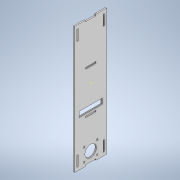
# Autodesk Inventor part: MuurL
Saved by Autodesk Inventor 2020 (Build 240168000, 168)
## iProperties
Created: 2020-01-30
Part Number: MuurL
Material: Generic
Document SubType Name: Modeling
Designer: jelte
Density: 1 g/cm^3
Appearance: Default
Mass: 62.7355 g
Surface Area: 455.02 cm^2
Volume: 62.7355 cm^3
Author: jelte
Autodesk Inventor part; units mm, degrees
ref_plane "YZ Plane" through (0, 0, 0) normal (1, 0, 0) x (0, 1, 0)
ref_plane "XZ Plane" through (0, 0, 0) normal (0, 1, 0) x (-1, 0, 0)
ref_plane "XY Plane" through (0, 0, 0) normal (0, 0, 1) x (1, 0, 0)
sketch "Sketch1" plane through (0, 0, 0) normal (1, 0, 0) x (0, 1, 0)
  line L0 (136.2492, 38.7083) -> (-163.7508, 38.7083)
  line L1 (-163.7508, -36.2917) -> (136.2492, -36.2917)
  line L2 (-160.7508, 13.7083) -> (-160.7508, -11.2917)
  line L3 (-160.7508, -11.2917) -> (-163.7508, -11.2917)
  line L4 (-160.7508, 13.7083) -> (-163.7508, 13.7083)
  line L5 (-163.7508, 13.7083) -> (-163.7508, 38.7083)
  line L6 (-163.7508, -11.2917) -> (-163.7508, -36.2917)
  line L7 (136.2492, 38.7083) -> (136.2492, 13.7083)
  line L8 (136.2492, -36.2917) -> (136.2492, -11.2917)
  line L9 (136.2492, 13.7083) -> (133.2492, 13.7083)
  line L10 (133.2492, 13.7083) -> (133.2492, -11.2917)
  line L11 (136.2492, -11.2917) -> (133.2492, -11.2917)
  point P0 (0, 0)
  dimension "d1" = 300
  constraints: 24 end point, 4 vertical, 2 equal length, 2 horizontal, 1 perpendicular
  measures "d1" distance of L1.start L1.end
extrude "Extrusion1" add sketch "Sketch1" along normal blind 3
sketch "Sketch2" plane through (3, 0, 0) normal (1, 0, 0) x (0, 0, -1)
  line L0 (-13.7083, -163.7508) -> (-13.7083, -160.7508) projected
  line L1 (-13.7083, -160.7508) -> (11.2917, -160.7508) projected
  line L2 (-13.7083, -60.7508) -> (11.2917, -60.7508)
  line L3 (11.2917, -60.7508) -> (11.2917, -63.7508)
  line L4 (11.2917, -63.7508) -> (-13.7083, -63.7508)
  line L5 (-13.7083, -63.7508) -> (-13.7083, -60.7508)
  line L6 (36.2917, -163.7508) -> (36.2917, 136.2492) projected
  line L7 (-13.7083, 36.2492) -> (11.2917, 36.2492)
  line L8 (11.2917, 36.2492) -> (11.2917, 39.2492)
  line L9 (11.2917, 39.2492) -> (-13.7083, 39.2492)
  line L10 (-13.7083, 39.2492) -> (-13.7083, 36.2492)
  point P0 (0, 0)
  constraints: 16 end point, 4 parallel, 2 horizontal, 2 perpendicular
extrude "Extrusion2" cut sketch "Sketch2" against normal blind 3
sketch "Sketch3" plane through (3, 0, 0) normal (1, 0, 0) x (0, 0, -1)
  line L0 (-13.7083, -160.7508) -> (11.2917, -160.7508) projected
  circle A0 centre (-16.7083, -154.7508) radius 1.5
  circle A1 centre (14.2917, -154.7508) radius 1.5
  circle A2 centre (14.2917, -123.7508) radius 1.5
  circle A3 centre (-16.7083, -123.7508) radius 1.5
  circle A4 centre (-1.2083, -139.2508) radius 12
  point P0 (0, 0)
  dimension "d29" = 3
  dimension "d30" = 3
  dimension "d31" = 3
  dimension "d32" = 3
  dimension "d33" = 24
  constraints: 5 centre point
  measures "d29" diameter of A2
  measures "d30" diameter of A3
  measures "d31" diameter of A0
  measures "d32" diameter of A1
  measures "d33" diameter of A4
extrude "Extrusion3" cut sketch "Sketch3" against normal blind 3
sketch "Sketch4" plane through (3, 0, 0) normal (1, 0, 0) x (0, 0, -1)
  line L0 (-13.7083, -160.7508) -> (11.2917, -160.7508) projected
  line L1 (36.2917, -163.7508) -> (36.2917, 136.2492) projected
  line L2 (31.2917, -155.7508) -> (28.2917, -155.7508)
  line L3 (28.2917, -155.7508) -> (28.2917, -145.7508)
  line L4 (28.2917, -145.7508) -> (31.2917, -145.7508)
  line L5 (31.2917, -145.7508) -> (31.2917, -155.7508)
  line L6 (-38.7083, 136.2492) -> (-38.7083, -163.7508) projected
  line L7 (-33.7083, -155.7508) -> (-30.7083, -155.7508)
  line L8 (-30.7083, -155.7508) -> (-30.7083, -145.7508)
  line L9 (-30.7083, -145.7508) -> (-33.7083, -145.7508)
  line L10 (-33.7083, -145.7508) -> (-33.7083, -155.7508)
  line L11 (-33.7083, 128.1373) -> (-30.7083, 128.1373)
  line L12 (-30.7083, 128.1373) -> (-30.7083, 118.1373)
  line L13 (-30.7083, 118.1373) -> (-33.7083, 118.1373)
  line L14 (-33.7083, 118.1373) -> (-33.7083, 128.1373)
  line L15 (31.2917, 128.1373) -> (28.2917, 128.1373)
  line L16 (28.2917, 128.1373) -> (28.2917, 118.1373)
  line L17 (28.2917, 118.1373) -> (31.2917, 118.1373)
  line L18 (31.2917, 118.1373) -> (31.2917, 128.1373)
  point P0 (0, 0)
  dimension "d38" = 3
  dimension "d39" = 10
  dimension "d46" = 3
  dimension "d47" = 10
  dimension "d48" = 3
  dimension "d49" = 10
  dimension "d50" = 10
  dimension "d51" = 3
  constraints: 32 end point, 8 parallel, 4 horizontal, 4 perpendicular
  measures "d38" distance of L3.end L4.end
  measures "d39" distance of L4.end L2.start
  measures "d46" distance of L8.end L9.end
  measures "d47" distance of L7.end L8.end
  measures "d48" distance of L12.end L13.end
  measures "d49" distance of L11.end L12.end
  measures "d50" distance of L15.end L16.end
  measures "d51" distance of L16.end L17.end
extrude "Extrusion4" cut sketch "Sketch4" against normal blind 30
sketch "Sketch5" plane through (3, 0, 0) normal (1, 0, 0) x (0, 0, -1)
  line L0 (-13.7083, -60.7508) -> (11.2917, -60.7508) projected
  line L1 (-38.7083, 136.2492) -> (-38.7083, -163.7508) projected
  line L2 (36.2917, -163.7508) -> (36.2917, 136.2492) projected
  line L3 (-28.7083, -55.7508) -> (26.2917, -55.7508)
  line L4 (26.2917, -55.7508) -> (26.2917, -43.2508)
  line L5 (26.2917, -43.2508) -> (-28.7083, -43.2508)
  line L6 (-28.7083, -43.2508) -> (-28.7083, -55.7508)
  point P0 (0, 0)
  constraints: 8 end point, 2 parallel, 1 horizontal, 1 perpendicular
extrude "Extrusion5" cut sketch "Sketch5" against normal blind 10
sketch "Sketch6" plane through (3, 0, 0) normal (1, 0, 0) x (0, 0, -1)
  line L0 (-30.7083, 118.1373) -> (-33.7083, 118.1373) projected
  line L1 (-33.7083, 118.1373) -> (-30.7083, 118.1373)
  line L2 (-30.7083, 118.1373) -> (-30.7083, 103.1373)
  line L3 (-30.7083, 103.1373) -> (-33.7083, 103.1373)
  line L4 (-33.7083, 103.1373) -> (-33.7083, 118.1373)
  line L5 (28.2917, 118.1373) -> (31.2917, 118.1373) projected
  line L6 (28.2917, 118.1373) -> (31.2917, 118.1373)
  line L7 (31.2917, 118.1373) -> (31.2917, 103.1373)
  line L8 (31.2917, 103.1373) -> (28.2917, 103.1373)
  line L9 (28.2917, 103.1373) -> (28.2917, 118.1373)
  line L10 (-33.7083, -155.7508) -> (-33.7083, -145.7508) projected
  line L11 (-33.7083, -145.7508) -> (-30.7083, -145.7508)
  line L12 (-30.7083, -145.7508) -> (-30.7083, -130.7508)
  line L13 (-30.7083, -130.7508) -> (-33.7083, -130.7508)
  line L14 (-33.7083, -130.7508) -> (-33.7083, -145.7508)
  line L15 (28.2917, -155.7508) -> (28.2917, -145.7508) projected
  line L16 (28.2917, -145.7508) -> (31.2917, -145.7508)
  line L17 (31.2917, -145.7508) -> (31.2917, -130.7508)
  line L18 (31.2917, -130.7508) -> (28.2917, -130.7508)
  line L19 (28.2917, -130.7508) -> (28.2917, -145.7508)
  point P0 (0, 0)
  dimension "d62" = 15
  dimension "d63" = 15
  constraints: 32 end point, 8 parallel, 4 horizontal, 4 perpendicular
  measures "d62" distance of L11.end L12.end
  measures "d63" distance of L16.end L17.end
extrude "Extrusion6" cut sketch "Sketch6" against normal blind 10
sketch "Sketch7" plane through (3, 0, 0) normal (1, 0, 0) x (0, 0, -1)
  point P0 (0, 0)
sketch "Sketch8" plane through (3, 0, 0) normal (1, 0, 0) x (0, 0, -1)
  circle A0 centre (-16.7083, -123.7508) radius 1.5 projected
  circle A1 centre (14.2917, -123.7508) radius 1.5 projected
  line L0 (-16.7083, -123.7508) -> (14.2917, -123.7508)
  circle A2 centre (14.2917, -154.7508) radius 1.5 projected
  line L1 (14.2917, -123.7508) -> (14.2917, -154.7508)
  circle A3 centre (-16.7083, -154.7508) radius 1.5 projected
  line L2 (14.2917, -154.7508) -> (-16.7083, -154.7508)
  line L3 (-16.7083, -154.7508) -> (-16.7083, -123.7508)
  circle A4 centre (-16.7083, -123.7508) radius 1.5
  circle A5 centre (14.2917, -123.7508) radius 1.5
  circle A6 centre (14.2917, -154.7508) radius 1.5
  circle A7 centre (-16.7083, -154.7508) radius 1.5
  circle A8 centre (-1.2083, -139.2508) radius 12 projected
  circle A9 centre (-1.2083, -139.2508) radius 12
  point P0 (0, 0)
  constraints: 8 end point, 5 centre point, 5 coincident, 4 concentric, 3 perpendicular, 1 horizontal
extrude "Extrusion7" add sketch "Sketch8" against normal blind 3 contours L0 L3 A0 | A0 L3 L0 | L0 L1 A1 | A1 L1 L0 | L3 L2 A3 | A3 L2 L3 | L1 L2 A2 | A2 L2 L1 | A8
sketch "Sketch9" plane through (3, 0, 0) normal (1, 0, 0) x (0, 0, -1)
  line L0 (11.2917, -163.7508) -> (36.2917, -163.7508) projected
  line L1 (-38.7083, -163.7508) -> (-13.7083, -163.7508) projected
  line L2 (36.2917, -163.7508) -> (36.2917, 136.2492) projected
  circle A0 centre (-16.7083, -153.7508) radius 2
  circle A1 centre (14.2917, -153.7508) radius 2
  circle A2 centre (14.2917, -122.7508) radius 2
  circle A3 centre (-16.7083, -122.7508) radius 2
  circle A4 centre (-1.2083, -138.2508) radius 12
  point P0 (0, 0)
  dimension "d75" = 4
  dimension "d76" = 4
  dimension "d77" = 4
  dimension "d78" = 4
  dimension "d79" = 24
  constraints: 5 centre point
  measures "d75" diameter of A3
  measures "d76" diameter of A2
  measures "d77" diameter of A1
  measures "d78" diameter of A0
  measures "d79" diameter of A4
extrude "Extrusion8" cut sketch "Sketch9" against normal blind 3
sketch "Sketch10" plane through (3, 0, 0) normal (1, 0, 0) x (0, 0, -1)
  circle A0 centre (-1.2083, -138.2508) radius 12 projected
  circle A1 centre (-1.2083, -138.2508) radius 13.75
  point P0 (0, 0)
  dimension "d82" = 27.5
  constraints: 1 centre point, 1 coincident
  measures "d82" diameter of A1
extrude "Extrusion9" cut sketch "Sketch10" against normal blind 10 contours A0 | A1
body "Solid1"
